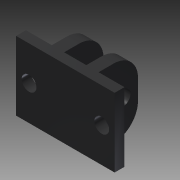
# Autodesk Inventor part: Part3
Saved by Autodesk Inventor 2016 (Build 200138000, 138)
## iProperties
Created: 2015-06-07
Part Number: Part3
Material: ABS Plastic
Document SubType Name: Modeling
Designer: Jufo
Density: 1 g/cm^3
Appearance: Smooth - White
Author: Jufo
Autodesk Inventor part; units mm, degrees
ref_plane "YZ Plane" through (0, 0, 0) normal (1, 0, 0) x (0, 1, 0)
ref_plane "XZ Plane" through (0, 0, 0) normal (0, 1, 0) x (-1, 0, 0)
ref_plane "XY Plane" through (0, 0, 0) normal (0, 0, 1) x (1, 0, 0)
sketch "Sketch1" plane through (0, 0, 0) normal (0, 1, 0) x (-1, 0, 0)
  line L0 (-2.8391, 8.5286) -> (6.6609, 8.5286)
  line L1 (6.6609, 8.5286) -> (6.6609, -5.4714)
  line L2 (-2.8391, 8.5286) -> (-2.8391, -5.4714)
  line L3 (-2.8391, -5.4714) -> (6.6609, -5.4714)
  line L4 (-0.3391, 8.5286) -> (-0.3391, -5.4714)
  line L5 (4.1609, 8.5286) -> (4.1609, -5.4714)
  line L6 (-2.8391, 8.5286) -> (-8.0891, 8.5286)
  line L7 (-8.0891, 8.5286) -> (-8.0891, -5.4714)
  line L8 (-8.0891, -5.4714) -> (-2.8391, -5.4714)
  line L9 (6.6609, 8.5286) -> (11.9109, 8.5286)
  line L10 (11.9109, 8.5286) -> (11.9109, -5.4714)
  line L11 (11.9109, -5.4714) -> (6.6609, -5.4714)
  circle A0 centre (-5.4641, 1.5286) radius 1.5
  circle A1 centre (9.2859, 1.5286) radius 1.5
  point P0 (0, 0)
  dimension "d0" = 4.5
  dimension "d3" = 2.5
  dimension "d5" = 2.5
  dimension "d7" = 20
  dimension "d8" = 5.25
  dimension "d9" = 5.25
  dimension "d10" = 14
  dimension "d11" = 3
  dimension "d12" = 3
  dimension "d27" = 2.625
  dimension "d28" = 2.625
  constraints: 24 end point, 6 perpendicular, 4 parallel, 4 point on line, 2 centre point, 1 horizontal
  measures "d0" distance between parallel lines of L5 L4
  measures "d3" distance between parallel lines of L1 L5
  measures "d5" distance between parallel lines of L2 L4
  measures "d7" distance between parallel lines of L7 L10
  measures "d8" distance of L7.end L2.end
  measures "d9" distance of L10.end L1.end
  measures "d10" distance of L9.end L10.end
  measures "d11" diameter of A0
  measures "d12" diameter of A1
  measures "d27" distance from line of L2 A0.centre
  measures "d28" distance from line of L1 A1.centre
extrude "Extrusion1" add sketch "Sketch1" along normal blind 2
sketch "Sketch2" plane through (0, 2, 0) normal (0, 1, 0) x (1, 0, 0)
  line L0 (8.0891, 5.4714) -> (-11.9109, 5.4714) projected
  line L1 (-11.9109, -8.5286) -> (8.0891, -8.5286) projected
  line L2 (-4.1609, 5.4714) -> (-4.1609, -8.5286)
  line L3 (-4.1609, -8.5286) -> (0.3391, -8.5286)
  line L4 (0.3391, -8.5286) -> (0.3391, 5.4714)
  line L5 (0.3391, 5.4714) -> (2.8391, 5.4714)
  line L6 (2.8391, 5.4714) -> (2.8391, -8.5286)
  line L7 (-6.6609, 5.4714) -> (-6.6609, -8.5286)
  circle A0 centre (5.4641, -1.5286) radius 1.5 projected
  point P0 (0, 0)
  dimension "d16" = 4.5
  dimension "d17" = 2.5
  dimension "d18" = 2.5
  dimension "d29" = 2.625
  constraints: 12 end point, 8 point on line, 4 perpendicular
  measures "d16" distance of L2.end L3.end
  measures "d17" distance of L4.end L5.end
  measures "d18" distance between parallel lines of L2 L7
  measures "d29" distance from line of A0.centre L6
extrude "Extrusion2" add sketch "Sketch2" along normal blind 8 contours L6 L1 L4 L0 | L2 L1 L7 L0
fillet "Fillet1" radius 5 4 edges at (-5.4109, 10, -5.4714) (-5.4109, 10, 8.5286) (1.5891, 10, 8.5286) (1.5891, 10, -5.4714)
sketch "Sketch3" plane through (-6.6609, 2, -5.4714) normal (-1, 0, 0) x (0, 0, 1)
  line L0 (14, 0) -> (0, 0) projected
  circle A0 centre (7, 5) radius 1.5
  point P0 (5.4714, -2)
  dimension "d23" = 3
  dimension "d24" = 5
  constraints: 1 centre point
  measures "d23" diameter of A0
  measures "d24" distance from line of L0 A0.centre
extrude "Extrusion3" cut sketch "Sketch3" against normal blind 20
body "Solid1"
